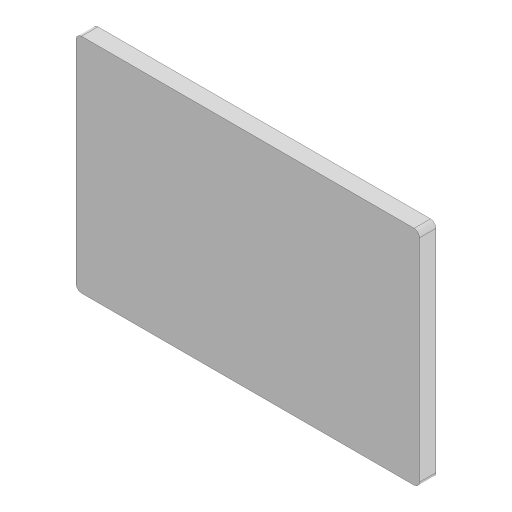
# Autodesk Inventor part: LaptopScaleModel
Saved by Autodesk Inventor 2024 (Build 280153000, 153)
## iProperties
Created: 2025-11-23
Part Number: LaptopScaleModel
Material: Generic
Document SubType Name: Modeling
Designer: gaoet
Density: 1 g/cm^3
Appearance: Default
Author: gaoet
Autodesk Inventor part; units mm, degrees
ref_plane "YZ Plane" through (0, 0, 0) normal (1, 0, 0) x (0, 1, 0)
ref_plane "XZ Plane" through (0, 0, 0) normal (0, 1, 0) x (-1, 0, 0)
ref_plane "XY Plane" through (0, 0, 0) normal (0, 0, 1) x (1, 0, 0)
sketch "Sketch1" plane through (0, 0, 0) normal (0, 0, 1) x (1, 0, 0)
  line L0 (200.025, -129.54) -> (-200.025, -129.54)
  line L1 (-200.025, -129.54) -> (-200.025, 129.54)
  line L2 (-200.025, 129.54) -> (200.025, 129.54)
  line L3 (200.025, 129.54) -> (200.025, -129.54)
  line L4 (200.025, -129.54) -> (-200.025, 129.54) construction
  line L5 (-200.025, -129.54) -> (200.025, 129.54) construction
  point P0 (0, 0)
  dimension "d0" = 400.05
  dimension "d1" = 259.08
  constraints: 12 end point, 2 midpoint, 2 parallel, 1 horizontal, 1 perpendicular
  measures "d0" distance of L1.end L2.end
  measures "d1" distance of L0.end L1.end
extrude "Extrusion1" add sketch "Sketch1" along normal blind 19.05
fillet "Fillet1" radius 6.35 4 edges at (-200.025, 129.54, 9.525) (200.025, 129.54, 9.525) (200.025, -129.54, 9.525) (-200.025, -129.54, 9.525)
body "Solid1"
